Autodesk Inventor part; units mm, degrees
(part 2 of 2)
sketch "Skizze21" plane through (-54.5, -24.5, 2.5) normal (-1, 0, 0) x (0, 0, 1)
  line L0 (-17.5, 17.5) -> (-2.5, 17.5) construction
  line L1 (-17.5, 25.5) -> (-17.5, 17.5) construction
  line L2 (-17.5, 25.5) -> (-2.5, 25.5) construction
  line L3 (0, 0) -> (-17, 0) construction
  line L4 (0, 0) -> (0, 64) construction
  line L5 (0, 64) -> (-17, 64) construction
  line L6 (-17, 0) -> (-17, 64) construction
  line L7 (-10.2358, 1.0735) -> (-3.5468, 1.0735) construction
  line L8 (-10.2358, 1.0735) -> (-4.1448, 2.982) construction
  line L9 (-4.1448, 2.982) -> (-3.5468, 1.0735) construction
  line L10 (-3.8371, 62) -> (-7.279, 62) construction
  line L11 (-3.8371, 62) -> (-3.5468, 61.0735) construction
  line L12 (-3.5468, 61.0735) -> (-14.9363, 57.5048) construction
  line L13 (-14.9363, 57.5048) -> (-15.5343, 59.4133) construction
  line L14 (-15.5343, 59.4133) -> (-7.279, 62) construction
  line L15 (-3.5468, 9.0735) -> (-14.9363, 5.5048) construction
  line L16 (-14.9363, 5.5048) -> (-15.5343, 7.4133) construction
  line L17 (-15.5343, 7.4133) -> (-4.1448, 10.982) construction
  line L18 (-4.1448, 10.982) -> (-3.5468, 9.0735) construction
  line L19 (-3.5468, 17.0735) -> (-14.9363, 13.5048) construction
  line L20 (-14.9363, 13.5048) -> (-15.5343, 15.4133) construction
  line L21 (-15.5343, 15.4133) -> (-4.1448, 18.982) construction
  line L22 (-4.1448, 18.982) -> (-3.5468, 17.0735) construction
  line L23 (-3.5468, 25.0735) -> (-14.9363, 21.5048) construction
  line L24 (-14.9363, 21.5048) -> (-15.5343, 23.4133) construction
  line L25 (-15.5343, 23.4133) -> (-4.1448, 26.982) construction
  line L26 (-4.1448, 26.982) -> (-3.5468, 25.0735) construction
  line L27 (-3.5468, 33.0735) -> (-14.9363, 29.5048) construction
  line L28 (-14.9363, 29.5048) -> (-15.5343, 31.4133) construction
  line L29 (-15.5343, 31.4133) -> (-4.1448, 34.982) construction
  line L30 (-4.1448, 34.982) -> (-3.5468, 33.0735) construction
  line L31 (-3.5468, 41.0735) -> (-14.9363, 37.5048) construction
  line L32 (-14.9363, 37.5048) -> (-15.5343, 39.4133) construction
  line L33 (-15.5343, 39.4133) -> (-4.1448, 42.982) construction
  line L34 (-4.1448, 42.982) -> (-3.5468, 41.0735) construction
  line L35 (-3.5468, 49.0735) -> (-14.9363, 45.5048) construction
  line L36 (-14.9363, 45.5048) -> (-15.5343, 47.4133) construction
  line L37 (-15.5343, 47.4133) -> (-4.1448, 50.982) construction
  line L38 (-4.1448, 50.982) -> (-3.5468, 49.0735) construction
  line L39 (-3.5468, 57.0735) -> (-14.9363, 53.5048) construction
  line L40 (-14.9363, 53.5048) -> (-15.5343, 55.4133) construction
  line L41 (-15.5343, 55.4133) -> (-4.1448, 58.982) construction
  line L42 (-4.1448, 58.982) -> (-3.5468, 57.0735) construction
  line L43 (-3.5468, 53.0735) -> (-14.9363, 49.5048) construction
  line L44 (-14.9363, 49.5048) -> (-15.5343, 51.4133) construction
  line L45 (-15.5343, 51.4133) -> (-4.1448, 54.982) construction
  line L46 (-4.1448, 54.982) -> (-3.5468, 53.0735) construction
  line L47 (-3.5468, 45.0735) -> (-14.9363, 41.5048) construction
  line L48 (-14.9363, 41.5048) -> (-15.5343, 43.4133) construction
  line L49 (-15.5343, 43.4133) -> (-4.1448, 46.982) construction
  line L50 (-4.1448, 46.982) -> (-3.5468, 45.0735) construction
  line L51 (-3.5468, 37.0735) -> (-14.9363, 33.5048) construction
  line L52 (-14.9363, 33.5048) -> (-15.5343, 35.4133) construction
  line L53 (-15.5343, 35.4133) -> (-4.1448, 38.982) construction
  line L54 (-4.1448, 38.982) -> (-3.5468, 37.0735) construction
  line L55 (-3.5468, 29.0735) -> (-14.9363, 25.5048) construction
  line L56 (-14.9363, 25.5048) -> (-15.5343, 27.4133) construction
  line L57 (-15.5343, 27.4133) -> (-4.1448, 30.982) construction
  line L58 (-4.1448, 30.982) -> (-3.5468, 29.0735) construction
  line L59 (-3.5468, 21.0735) -> (-14.9363, 17.5048) construction
  line L60 (-14.9363, 17.5048) -> (-15.5343, 19.4133) construction
  line L61 (-15.5343, 19.4133) -> (-4.1448, 22.982) construction
  line L62 (-4.1448, 22.982) -> (-3.5468, 21.0735) construction
  line L63 (-3.5468, 13.0735) -> (-14.9363, 9.5048) construction
  line L64 (-14.9363, 9.5048) -> (-15.5343, 11.4133) construction
  line L65 (-15.5343, 11.4133) -> (-4.1448, 14.982) construction
  line L66 (-4.1448, 14.982) -> (-3.5468, 13.0735) construction
  line L67 (-3.5468, 5.0735) -> (-14.9363, 1.5048) construction
  line L68 (-14.9363, 1.5048) -> (-15.5343, 3.4133) construction
  line L69 (-15.5343, 3.4133) -> (-4.1448, 6.982) construction
  line L70 (-4.1448, 6.982) -> (-3.5468, 5.0735) construction
  line L71 (0, 0) -> (0, 64) construction
  line L72 (0, 25.5048) -> (-17, 25.5048) construction
  line L73 (-17, 25.5048) -> (-17, 17.5) construction
  line L74 (-17, 17.5) -> (0, 17.5) construction
  line L75 (0, 17.5) -> (0, 25.5048) construction
  line L76 (-2, 60.1804) -> (-2, 1.6) construction
  line L77 (-2, 25.5048) -> (-2, 30.0048) construction
  line L78 (-17, -13) -> (-17, 62) projected
  line L79 (0, 30.0048) -> (-17, 30.0048)
  line L80 (-17, 30.0048) -> (-17, 36.0048)
  line L81 (-17, 36.0048) -> (0, 36.0048)
  line L82 (0, 36.0048) -> (0, 30.0048)
  line L83 (0, 25.5048) -> (-17, 25.5048)
  line L84 (-17, 25.5048) -> (-17, 19.5048)
  line L85 (-17, 19.5048) -> (0, 19.5048)
  line L86 (0, 19.5048) -> (0, 25.5048)
  point P0 (-2.5, 24.5)
  dimension "d146" = 4.5
  dimension "d147" = 6
  dimension "d148" = 6
  constraints: 30 end point, 9 point on line, 6 parallel, 5 horizontal, 3 perpendicular, 3 other
  measures "d146" distance of L77.start L77.end
  measures "d147" distance of L79.end L80.end
  measures "d148" distance of L84.end L83.end
extrude "Extrusion24" add sketch "Skizze21" along normal blind 10 from surface at -2
sketch "Skizze22" plane through (0, 0, -14.5) normal (0, 0, -1) x (-1, 0, 0)
  line L0 (54.5, -4.9952) -> (62.5, -4.9952) construction
  line L1 (62.5, 1.0048) -> (62.5, -4.9952) construction
  line L2 (54.5, 1.0048) -> (62.5, 1.0048) construction
  line L3 (62.5, 5.5048) -> (54.5, 5.5048) construction
  line L4 (62.5, 11.5048) -> (62.5, 5.5048) construction
  line L5 (62.5, 11.5048) -> (54.5, 11.5048) construction
  line L6 (54.5, 11.5048) -> (54.5, 39.5) construction
  line L7 (62.5, 1.0048) -> (62.5, -4.9952) construction
  line L8 (54.5, 1.0048) -> (62.5, 1.0048) construction
  line L9 (54.5, 1.0048) -> (54.5, 5.5048) construction
  line L10 (62.5, 5.5048) -> (54.5, 5.5048) construction
  line L11 (62.5, 11.5048) -> (62.5, 5.5048) construction
  line L12 (62.5, 11.5048) -> (54.5, 11.5048) construction
  line L13 (54.5, 11.5048) -> (54.5, 39.5) construction
  line L14 (54.5, 39.5) -> (-54.5, 39.5) construction
  line L15 (-54.5, 39.5) -> (-54.5, -39.5) construction
  line L16 (-54.5, -39.5) -> (9.5, -39.5) construction
  line L17 (9.5, -39.5) -> (9.5, -37.5) construction
  line L18 (9.5, -37.5) -> (-52.5, -37.5) construction
  line L19 (-52.5, -37.5) -> (-52.5, 37.5) construction
  line L20 (-52.5, 37.5) -> (52.5, 37.5) construction
  line L21 (52.5, 37.5) -> (52.5, -24.5) construction
  line L22 (52.5, -24.5) -> (54.5, -24.5) construction
  line L23 (54.5, -24.5) -> (54.5, -4.9952) construction
  line L24 (54.5, -4.9952) -> (62.5, -4.9952) construction
  line L25 (62.5, -4.9952) -> (52.5, -4.9952)
  line L26 (52.5, -4.9952) -> (52.5, 1.0048)
  line L27 (52.5, 1.0048) -> (62.5, 1.0048)
  line L28 (62.5, 1.0048) -> (62.5, -4.9952)
  line L29 (62.5, 5.5048) -> (52.5, 5.5048)
  line L30 (52.5, 5.5048) -> (52.5, 11.5048)
  line L31 (52.5, 11.5048) -> (62.5, 11.5048)
  line L32 (62.5, 11.5048) -> (62.5, 5.5048)
  point P0 (0, 0)
  constraints: 16 end point, 4 parallel, 2 horizontal, 2 perpendicular, 2 point on line
extrude "Extrusion25" add sketch "Skizze22" along normal blind 10
sketch "Skizze23" plane through (0, 0, 2.5) normal (0, 0, 1) x (1, 0, 0)
  line L0 (-41.5, 35.6804) -> (-41.5, -22.9) construction
  line L1 (-41.5, -22.9) -> (-43.9777, -22.9) construction
  line L2 (-43.9777, -22.9) -> (-43.9777, 35.6804) construction
  line L3 (-43.9777, 35.6804) -> (-41.5, 35.6804) construction
  line L4 (-54.5, -24.5) -> (-32.8176, -24.5) construction
  arc A0 (-32.8176, -24.5) -> (-11.4624, -29.9989) centre (-10.5668, 17.6958) ccw construction
  arc A1 (-9.5, -31.9985) -> (-11.4624, -29.9989) centre (-11.5, -31.9985) ccw construction
  line L5 (-9.5, -31.9985) -> (-9.5, -39.5) construction
  line L6 (54.5, -39.5) -> (-9.5, -39.5) construction
  line L7 (54.5, 39.5) -> (54.5, -39.5) construction
  line L8 (-54.5, 39.5) -> (54.5, 39.5) construction
  line L9 (-54.5, 11.5048) -> (-54.5, 39.5) construction
  line L10 (-62.5, 11.5048) -> (-54.5, 11.5048) construction
  line L11 (-62.5, 5.5048) -> (-62.5, 11.5048) construction
  line L12 (-54.5, 5.5048) -> (-62.5, 5.5048) construction
  line L13 (-54.5, 1.0048) -> (-54.5, 5.5048) construction
  line L14 (-62.5, 1.0048) -> (-54.5, 1.0048) construction
  line L15 (-62.5, -4.9952) -> (-62.5, 1.0048) construction
  line L16 (-54.5, -4.9952) -> (-62.5, -4.9952) construction
  line L17 (-54.5, -24.5) -> (-54.5, -4.9952) construction
  line L18 (-47.5, 35.6804) -> (-47.5, -0.041) construction
  line L19 (-47.5, -0.041) -> (-49.9777, -0.041) construction
  line L20 (-49.9777, -0.041) -> (-49.9777, 35.6804) construction
  line L21 (-49.9777, 35.6804) -> (-47.5, 35.6804) construction
  circle A2 centre (-47.5, -3) radius 1.35 construction
  line L22 (36.5, 27.1) -> (36.5, -35.7623) construction
  line L23 (36.5, -35.7623) -> (34.0223, -35.7623) construction
  line L24 (34.0223, -35.7623) -> (34.0223, 27.1) construction
  line L25 (34.0223, 27.1) -> (36.5, 27.1) construction
  line L26 (30.5, -25.9706) -> (30.5, -35.7623) construction
  line L27 (30.5, -35.7623) -> (28.0223, -35.7623) construction
  line L28 (28.0223, -35.7623) -> (28.0223, -25.9706) construction
  line L29 (28.0223, -25.9706) -> (30.5, -25.9706) construction
  line L30 (18.5, -28.5) -> (18.5, -35.7623) construction
  line L31 (18.5, -35.7623) -> (16.0223, -35.7623) construction
  line L32 (16.0223, -35.7623) -> (16.0223, -28.5) construction
  line L33 (16.0223, -28.5) -> (18.5, -28.5) construction
  line L34 (-29.5, -16.7561) -> (-29.5, -22.9) construction
  line L35 (-29.5, -22.9) -> (-31.9777, -22.9) construction
  line L36 (-31.9777, -22.9) -> (-31.9777, -16.7561) construction
  line L37 (-31.9777, -16.7561) -> (-29.5, -16.7561) construction
  line L38 (-25.9777, 30.1243) -> (-25.9777, 35.6804) construction
  line L39 (-25.9777, 35.6804) -> (-23.5, 35.6804) construction
  line L40 (-23.5, 35.6804) -> (-23.5, 30.1243) construction
  line L41 (-23.5, 30.1243) -> (-25.9777, 30.1243) construction
  line L42 (16.0223, 31.6466) -> (16.0223, 35.6804) construction
  line L43 (16.0223, 35.6804) -> (18.5, 35.6804) construction
  line L44 (18.5, 35.6804) -> (18.5, 31.6466) construction
  line L45 (18.5, 31.6466) -> (16.0223, 31.6466) construction
  line L46 (-5.5, -32.1312) -> (-5.5, -35.7623) construction
  line L47 (-5.5, -35.7623) -> (-7.9777, -35.7623) construction
  line L48 (-7.9777, -35.7623) -> (-7.9777, -32.1312) construction
  line L49 (-7.9777, -32.1312) -> (-5.5, -32.1312) construction
  line L50 (10.0223, 32.8979) -> (10.0223, 35.6804) construction
  line L51 (10.0223, 35.6804) -> (12.5, 35.6804) construction
  line L52 (12.5, 35.6804) -> (12.5, 32.8979) construction
  line L53 (12.5, 32.8979) -> (10.0223, 32.8979) construction
  line L54 (-7.9777, 33.0955) -> (-7.9777, 35.6804) construction
  line L55 (-7.9777, 35.6804) -> (-5.5, 35.6804) construction
  line L56 (-5.5, 35.6804) -> (-5.5, 33.0955) construction
  line L57 (-5.5, 33.0955) -> (-7.9777, 33.0955) construction
  line L58 (0.5, -33.9467) -> (0.5, -35.7623) construction
  line L59 (0.5, -35.7623) -> (-1.9777, -35.7623) construction
  line L60 (-1.9777, -35.7623) -> (-1.9777, -33.9467) construction
  line L61 (-1.9777, -33.9467) -> (0.5, -33.9467) construction
  line L62 (-1.9777, 34.0902) -> (-1.9777, 35.6804) construction
  line L63 (-1.9777, 35.6804) -> (0.5, 35.6804) construction
  line L64 (0.5, 35.6804) -> (0.5, 34.0902) construction
  line L65 (0.5, 34.0902) -> (-1.9777, 34.0902) construction
  line L66 (6.5, -33.9467) -> (6.5, -35.7623) construction
  line L67 (6.5, -35.7623) -> (4.0223, -35.7623) construction
  line L68 (4.0223, -35.7623) -> (4.0223, -33.9467) construction
  line L69 (4.0223, -33.9467) -> (6.5, -33.9467) construction
  line L70 (4.0223, 32.8979) -> (4.0223, 35.6804) construction
  line L71 (4.0223, 35.6804) -> (6.5, 35.6804) construction
  line L72 (6.5, 35.6804) -> (6.5, 32.8979) construction
  line L73 (6.5, 32.8979) -> (4.0223, 32.8979) construction
  line L74 (-13.9777, 32.5) -> (-13.9777, 35.6804) construction
  line L75 (-13.9777, 35.6804) -> (-11.5, 35.6804) construction
  line L76 (-11.5, 35.6804) -> (-11.5, 32.5) construction
  line L77 (-11.5, 32.5) -> (-13.9777, 32.5) construction
  line L78 (12.5, -32.1312) -> (12.5, -35.7623) construction
  line L79 (12.5, -35.7623) -> (10.0223, -35.7623) construction
  line L80 (10.0223, -35.7623) -> (10.0223, -32.1312) construction
  line L81 (10.0223, -32.1312) -> (12.5, -32.1312) construction
  line L82 (-19.9777, 31.3064) -> (-19.9777, 35.6804) construction
  line L83 (-19.9777, 35.6804) -> (-17.5, 35.6804) construction
  line L84 (-17.5, 35.6804) -> (-17.5, 31.3064) construction
  line L85 (-17.5, 31.3064) -> (-19.9777, 31.3064) construction
  line L86 (22.0223, 30) -> (22.0223, 35.6804) construction
  line L87 (22.0223, 35.6804) -> (24.5, 35.6804) construction
  line L88 (24.5, 35.6804) -> (24.5, 30) construction
  line L89 (24.5, 30) -> (22.0223, 30) construction
  line L90 (-29.5, 27.1) -> (-29.5, 20.9081) construction
  line L91 (-29.5, 20.9081) -> (-31.9777, 20.9081) construction
  line L92 (-31.9777, 20.9081) -> (-31.9777, 27.1) construction
  line L93 (-31.9777, 27.1) -> (-29.5, 27.1) construction
  line L94 (24.5, -28.5) -> (24.5, -35.7623) construction
  line L95 (24.5, -35.7623) -> (22.0223, -35.7623) construction
  line L96 (22.0223, -35.7623) -> (22.0223, -28.5) construction
  line L97 (22.0223, -28.5) -> (24.5, -28.5) construction
  line L98 (-49.9777, -22.9) -> (-49.9777, -6.1402) construction
  line L99 (-49.9777, -6.1402) -> (-47.5, -6.1402) construction
  line L100 (-47.5, -6.1402) -> (-47.5, -22.9) construction
  line L101 (-47.5, -22.9) -> (-49.9777, -22.9) construction
  line L102 (46.0223, -27.1) -> (46.0223, 35.6804) construction
  line L103 (46.0223, 35.6804) -> (48.5, 35.6804) construction
  line L104 (48.5, 35.6804) -> (48.5, -27.1) construction
  line L105 (48.5, -27.1) -> (46.0223, -27.1) construction
  line L106 (40.0223, 35.6804) -> (42.5, 35.6804) construction
  line L107 (42.5, 35.6804) -> (42.5, -35.7623) construction
  line L108 (42.5, -35.7623) -> (40.0223, -35.7623) construction
  line L109 (40.0223, -35.7623) -> (40.0223, 35.6804) construction
  circle A3 centre (0, 0) radius 30 construction
  circle A4 centre (25, 25) radius 2.1 construction
  circle A5 centre (-25, 25) radius 2.1 construction
  circle A6 centre (-25, -25) radius 2.1 construction
  circle A7 centre (25, -25) radius 2.1 construction
  circle A8 centre (32, 32.5) radius 1.35 construction
  circle A9 centre (-30, 32.5) radius 1.35 construction
  circle A10 centre (47.5, -32.5) radius 1.35 construction
  line L110 (-35.5, 35.6804) -> (-35.5, -22.9) construction
  line L111 (-35.5, -22.9) -> (-37.9777, -22.9) construction
  line L112 (-37.9777, -22.9) -> (-37.9777, 35.6804) construction
  line L113 (-37.9777, 35.6804) -> (-35.5, 35.6804) construction
  line L114 (-54.5, 5.5048) -> (-62.5, 5.5048) projected
  line L115 (-62.5, 5.5048) -> (-54.5, 5.5048)
  line L116 (-54.5, 5.5048) -> (-54.5, 11.5048)
  line L117 (-54.5, 11.5048) -> (-62.5, 11.5048)
  line L118 (-62.5, 11.5048) -> (-62.5, 5.5048)
  line L119 (-54.5, 1.0048) -> (-54.5, 5.5048) projected
  line L120 (-62.5, -4.9952) -> (-54.5, -4.9952)
  line L121 (-54.5, -4.9952) -> (-54.5, 1.0048)
  line L122 (-54.5, 1.0048) -> (-62.5, 1.0048)
  line L123 (-62.5, 1.0048) -> (-62.5, -4.9952)
  constraints: 16 end point, 4 parallel, 2 horizontal, 2 perpendicular
extrude "Extrusion26" cut sketch "Skizze23" against normal blind 4
sketch "Skizze24" plane through (-54.5, -4.9952, -14.5) normal (0, -1, 0) x (1, 0, 0)
  line L0 (0, 13) -> (-8, 13) construction
  line L1 (-8, -10) -> (-8, 13) construction
  line L2 (2, -10) -> (-8, -10) construction
  line L3 (2, 0) -> (2, -10) construction
  line L4 (0, 0) -> (2, 0) construction
  line L5 (0, 1.7577) -> (0, 0) construction
  line L6 (2, 1.7577) -> (0, 1.7577) construction
  line L7 (2, 1.7577) -> (2, 8.4467) construction
  line L8 (0, 8.4467) -> (2, 8.4467) construction
  line L9 (0, 13) -> (0, 8.4467) construction
  circle A0 centre (-3, -3.7188) radius 1.75
  point P0 (54.5, 14.5)
  dimension "d155" = 3.5
  constraints: 1 centre point
  measures "d155" diameter of A0
extrude "Extrusion27" cut sketch "Skizze24" against normal through all
fillet "Rundung4" radius 2 14 edges at (-58.5, -4.9952, -1.5) (-58.5, 1.0048, -1.5) (-58.5, 5.5048, -1.5) (-58.5, 11.5048, -1.5) (-62.5, 8.5048, -1.5) (-62.5, -1.9952, -1.5) (-62.5, -4.9952, -13) (-62.5, 1.0048, -13) (-62.5, 5.5048, -13) (-62.5, 11.5048, -13) (-62.5, 8.5048, -24.5) (-62.5, -1.9952, -24.5) (-57.5, -4.9952, -24.5) (-57.5, 11.5048, -24.5)
fillet "Rundung5" radius 2 8 edges at (-54.5, 7.5, 2.5) (22.5, -39.5, 2.5) (54.5, 0, 2.5) (0, 39.5, 2.5) (54.5, -39.5, -6) (-54.5, -24.5, -6) (-54.5, 39.5, -6) (54.5, 39.5, -6)
fillet "Rundung6" radius 2 1 edges at (-30, 0, 2.5)
